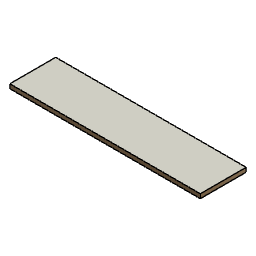
control_panel_bottom (Autodesk Fusion 360 design; units mm, degrees)
Autodesk Fusion 360 part; units mm, degrees
sketch "Control Panel Bottom" plane through (0, 0, 0) normal (0, 0, 1) x (1, 0, 0)
  line L0 (0, 0) -> (270, 0)
  line L1 (270, 0) -> (270, 65)
  line L2 (270, 65) -> (0, 65)
  line L3 (0, 65) -> (0, 0)
  dimension "d5" = 65
  dimension "d7" = 270
  constraint horizontal L0
  constraint vertical L1
  constraint horizontal L2
  constraint vertical L3
  constraint coincident L0.start L3.end
  measures "d5" distance of L0.end L1.end
  measures "d7" distance of L0.start L0.end
extrude "Extrude1" add sketch "Control Panel Bottom" along normal blind 6
equation "MDFThickness = 6 mm" comment "Thickness of the MDF board"
equation "d2 = MDFThickness"
equation "d5 = sidePanelControlPanelDepth"
equation "sidePanelControlPanelDepth = 65 mm" comment "Depth of the scontrol panel section of the side panel"
named bodies: "Control Panel Bottom"
